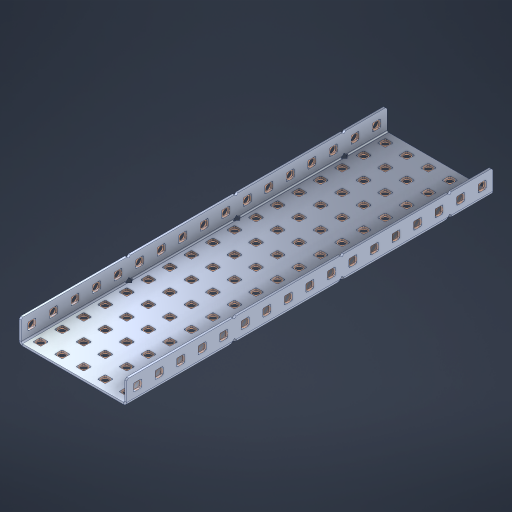
# Autodesk Inventor part: Alu C 1x3x1x35
Saved by Autodesk Inventor 2023 (Build 270158000, 158)
## iProperties
Created: 2022-07-28
Part Number: Alu C 1x3x1x35
Material: Generic
Document SubType Name: Sheet Metal
Designer: ylu12
Density: 1 g/cm^3
Sheet Metal Rule: Default
Appearance: Steel
Author: ylu12
Autodesk Inventor part; units mm, degrees
ref_plane "YZ Plane" through (0, 0, 0) normal (1, 0, 0) x (0, 1, 0)
ref_plane "XZ Plane" through (0, 0, 0) normal (0, 1, 0) x (-1, 0, 0)
sketch "Sketch1" plane through (0, 0, 0) normal (0, 1, 0) x (-1, 0, 0)
  line L0 (-31.75, 0) -> (31.75, 0)
  line L1 (31.75, 0) -> (31.75, -215.9)
  line L2 (31.75, -215.9) -> (-31.75, -215.9)
  line L3 (-31.75, -215.9) -> (-31.75, 0)
  line L4 (31.75, 0) -> (-31.75, -215.9) construction
  point P0 (0, 0)
  point P1 (0, 0)
  dimension "d0" = 63.5
  dimension "d1" = 215.9
  measures "d0" distance of L1.end L2.end
  measures "d1" distance of L0.end L1.end
extrude "Plate1" add sketch "Sketch1" along normal blind 1.1906
sketch "Sketch2" plane through (30.5594, 0, -215.9) normal (1, 0, 0) x (0, 1, 0)
  line L0 (0, 215.9) -> (0, 0)
  line L1 (0, 0) -> (13.8906, 0)
  line L2 (13.8906, 0) -> (13.8906, 215.9)
  line L3 (13.8906, 215.9) -> (0, 215.9)
  constraints: 6 end point, 1 horizontal, 1 perpendicular, 1 vertical
edge flange "Flanges" height 12.7 angle 90 thickness 1.1906 bend radius 0.7937 thickness toward (1, 0, 0) relief tear relief width 1.1906 relief depth 0.5953 corner gap 1.1906 corner form 0 edges at (31.75, 1.1906, -107.95) (-31.75, 1.1906, -107.95) wall of the first edge with corners at (30.5594, 0, 0) (30.5594, 0, -215.9) (30.5594, 13.8906, -215.9) (30.5594, 13.8906, 0)
bend "Bend1"
corner "Corner1"
sketch "Sketch3" plane through (31.75, 1.9844, -215.9) normal (1, 0, 0) x (0, 0, -1)
  line L0 (-211.3534, 7.8677) -> (-207.7466, 7.8677)
  line L1 (-207.2386, 7.3597) -> (-207.2386, 3.7529)
  line L2 (-207.7466, 3.2449) -> (-211.3534, 3.2449)
  line L3 (-211.8614, 3.7529) -> (-211.8614, 7.3597)
  arc A0 (-211.3534, 7.8677) -> (-211.8614, 7.3597) centre (-211.3534, 7.3597) ccw
  arc A1 (-207.2386, 7.3597) -> (-207.7466, 7.8677) centre (-207.7466, 7.3597) ccw
  arc A2 (-207.7466, 3.2449) -> (-207.2386, 3.7529) centre (-207.7466, 3.7529) ccw
  arc A3 (-211.8614, 3.7529) -> (-211.3534, 3.2449) centre (-211.3534, 3.7529) ccw
  line L4 (-215.9, 0) -> (-215.9, 11.9063) construction
  line L5 (-215.9, 11.9063) -> (0, 11.9063) construction
  line L6 (-211.3534, 7.3597) -> (-207.7466, 3.7529) construction
  point P0 (-215.9, -1.9844)
  point P1 (-207.2386, 3.2449)
  point P2 (-211.8614, 3.2449)
  point P3 (-209.55, 5.5563)
  dimension "d16" = 4.6228
  dimension "d17" = 0.508
  dimension "d20" = 6.35
  dimension "d21" = 6.35
  constraints: 10 end point, 8 point on circle, 8 tangent, 4 centre point, 4 point on line, 3 equal radius, 2 parallel, 2 perpendicular, 1 horizontal, 1 midpoint
  measures "d16" distance of point (-207.239, 3.245) point (-211.861, 3.245)
  measures "d17" radius of A0
  measures "d20" distance from line of point (-209.55, 5.556) L4
  measures "d21" distance from line of L5 point (-209.55, 5.556)
extrude "Flange Stamp" cut sketch "Sketch3" against normal blind 1.1906
sketch "Sketch7" plane through (31.75, 1.9844, 0) normal (1, 0, 0) x (0, 0, -1)
  arc A0 (4.5466, 7.8677) -> (4.0386, 7.3597) centre (4.5466, 7.3597) ccw construction
  arc A1 (8.1534, 3.2449) -> (8.6614, 3.7529) centre (8.1534, 3.7529) ccw construction
  circle A2 centre (6.35, 5.5563) radius 2.1844
  line L0 (4.5466, 7.3597) -> (8.1534, 3.7529) construction
  point P0 (0, -1.9844)
  dimension "d46" = 4.3688
  constraints: 2 end point, 1 centre point, 1 midpoint
  measures "d46" diameter of A2
surface extrude "Flange Circle" sketch "Sketch7" against normal up to surface (1.1906 mm away) shown yes curves A2
ref_plane "Flange Pattern Plane" through (31.75, 7.5406, -4.5466) normal (0, 1, 0) x (1, 0, 0)
pattern_sketch "Flange Pattern" of "Flange Circle", "Flange Stamp" from (31.75, 7.5406, -6.35) facing (1, 0, 0) copies at (31.75, 7.5406, -19.05) facing (1, 0, 0) at (31.75, 7.5406, -31.75) facing (1, 0, 0) at (31.75, 7.5406, -44.45) facing (1, 0, 0) at (31.75, 7.5406, -57.15) facing (1, 0, 0) at (31.75, 7.5406, -69.85) facing (1, 0, 0) at (31.75, 7.5406, -82.55) facing (1, 0, 0) at (31.75, 7.5406, -95.25) facing (1, 0, 0) at (31.75, 7.5406, -107.95) facing (1, 0, 0) at (31.75, 7.5406, -120.65) facing (1, 0, 0) at (31.75, 7.5406, -133.35) facing (1, 0, 0) at (31.75, 7.5406, -146.05) facing (1, 0, 0) at (31.75, 7.5406, -158.75) facing (1, 0, 0) at (31.75, 7.5406, -171.45) facing (1, 0, 0) at (31.75, 7.5406, -184.15) facing (1, 0, 0) at (31.75, 7.5406, -196.85) facing (1, 0, 0) at (31.75, 7.5406, -209.55) facing (1, 0, 0) at (-31.75, 7.5406, -6.35) facing (-1, 0, 0) at (-31.75, 7.5406, -19.05) facing (-1, 0, 0) at (-31.75, 7.5406, -31.75) facing (-1, 0, 0) at (-31.75, 7.5406, -44.45) facing (-1, 0, 0) at (-31.75, 7.5406, -57.15) facing (-1, 0, 0) at (-31.75, 7.5406, -69.85) facing (-1, 0, 0) at (-31.75, 7.5406, -82.55) facing (-1, 0, 0) at (-31.75, 7.5406, -95.25) facing (-1, 0, 0) at (-31.75, 7.5406, -107.95) facing (-1, 0, 0) at (-31.75, 7.5406, -120.65) facing (-1, 0, 0) at (-31.75, 7.5406, -133.35) facing (-1, 0, 0) at (-31.75, 7.5406, -146.05) facing (-1, 0, 0) at (-31.75, 7.5406, -158.75) facing (-1, 0, 0) at (-31.75, 7.5406, -171.45) facing (-1, 0, 0) at (-31.75, 7.5406, -184.15) facing (-1, 0, 0) at (-31.75, 7.5406, -196.85) facing (-1, 0, 0) at (-31.75, 7.5406, -209.55) facing (-1, 0, 0)
sketch "Sketch8" plane through (0, 0, 0) normal (0, -1, 0) x (1, 0, 0)
  line L0 (29.7656, 0) -> (-29.7656, 0) construction
  line L1 (27.2034, -4.0386) -> (23.5966, -4.0386)
  line L2 (23.0886, -4.5466) -> (23.0886, -8.1534)
  line L3 (23.5966, -8.6614) -> (27.2034, -8.6614)
  line L4 (27.7114, -8.1534) -> (27.7114, -4.5466)
  arc A0 (27.7114, -4.5466) -> (27.2034, -4.0386) centre (27.2034, -4.5466) ccw
  arc A1 (27.2034, -8.6614) -> (27.7114, -8.1534) centre (27.2034, -8.1534) ccw
  arc A2 (23.0886, -8.1534) -> (23.5966, -8.6614) centre (23.5966, -8.1534) ccw
  arc A3 (23.5966, -4.0386) -> (23.0886, -4.5466) centre (23.5966, -4.5466) ccw
  line L5 (27.2034, -4.5466) -> (23.5966, -8.1534) construction
  line L6 (31.75, 0) -> (31.75, -215.9) construction
  point P0 (0, 0)
  point P1 (23.0886, -8.6614)
  point P2 (27.7114, -8.6614)
  point P3 (25.4, -6.35)
  dimension "d49" = 4.6228
  dimension "d50" = 0.508
  dimension "d51" = 6.35
  dimension "d52" = 6.35
  constraints: 10 end point, 8 point on circle, 8 tangent, 4 centre point, 4 point on line, 3 equal radius, 2 parallel, 2 perpendicular, 1 horizontal, 1 midpoint
  measures "d49" distance of point (27.711, -8.661) point (23.089, -8.661)
  measures "d50" radius of A0
  measures "d51" distance from line of L6 point (25.4, -6.35)
  measures "d52" distance from line of L0 point (25.4, -6.35)
extrude "Body Stamp" cut sketch "Sketch8" against normal blind 1.1906
sketch "Sketch9" plane through (0, 0, 0) normal (0, -1, 0) x (1, 0, 0)
  arc A0 (27.7114, -4.5466) -> (27.2034, -4.0386) centre (27.2034, -4.5466) ccw construction
  arc A1 (23.0886, -8.1534) -> (23.5966, -8.6614) centre (23.5966, -8.1534) ccw construction
  line L0 (27.2034, -4.5466) -> (23.5966, -8.1534) construction
  circle A2 centre (25.4, -6.35) radius 2.1844
  point P0 (0, 0)
  dimension "d55" = 4.3688
  constraints: 2 end point, 1 centre point, 1 midpoint
  measures "d55" diameter of A2
surface extrude "Body Circle" sketch "Sketch9" against normal up to surface (1.1906 mm away) shown yes curves A2
pattern_sketch "Body Pattern" of "Body Stamp", "Body Circle" from (25.4, 0, -6.35) copies at (25.4, 0, -19.05) at (25.4, 0, -31.75) at (25.4, 0, -44.45) at (25.4, 0, -57.15) at (25.4, 0, -69.85) at (25.4, 0, -82.55) at (25.4, 0, -95.25) at (25.4, 0, -107.95) at (25.4, 0, -120.65) at (25.4, 0, -133.35) at (25.4, 0, -146.05) at (25.4, 0, -158.75) at (25.4, 0, -171.45) at (25.4, 0, -184.15) at (25.4, 0, -196.85) at (25.4, 0, -209.55) at (12.7, 0, -6.35) at (12.7, 0, -19.05) at (12.7, 0, -31.75) at (12.7, 0, -44.45) at (12.7, 0, -57.15) at (12.7, 0, -69.85) at (12.7, 0, -82.55) at (12.7, 0, -95.25) at (12.7, 0, -107.95) at (12.7, 0, -120.65) at (12.7, 0, -133.35) at (12.7, 0, -146.05) at (12.7, 0, -158.75) at (12.7, 0, -171.45) at (12.7, 0, -184.15) at (12.7, 0, -196.85) at (12.7, 0, -209.55) at (0, 0, -6.35) at (0, 0, -19.05) at (0, 0, -31.75) at (0, 0, -44.45) at (0, 0, -57.15) at (0, 0, -69.85) at (0, 0, -82.55) at (0, 0, -95.25) at (0, 0, -107.95) at (0, 0, -120.65) at (0, 0, -133.35) at (0, 0, -146.05) at (0, 0, -158.75) at (0, 0, -171.45) at (0, 0, -184.15) at (0, 0, -196.85) at (0, 0, -209.55) at (-12.7, 0, -6.35) at (-12.7, 0, -19.05) at (-12.7, 0, -31.75) at (-12.7, 0, -44.45) at (-12.7, 0, -57.15) at (-12.7, 0, -69.85) at (-12.7, 0, -82.55) at (-12.7, 0, -95.25) at (-12.7, 0, -107.95) at (-12.7, 0, -120.65) at (-12.7, 0, -133.35) at (-12.7, 0, -146.05) at (-12.7, 0, -158.75) at (-12.7, 0, -171.45) at (-12.7, 0, -184.15) at (-12.7, 0, -196.85) at (-12.7, 0, -209.55) at (-25.4, 0, -6.35) at (-25.4, 0, -19.05) at (-25.4, 0, -31.75) at (-25.4, 0, -44.45) at (-25.4, 0, -57.15) at (-25.4, 0, -69.85) at (-25.4, 0, -82.55) at (-25.4, 0, -95.25) at (-25.4, 0, -107.95) at (-25.4, 0, -120.65) at (-25.4, 0, -133.35) at (-25.4, 0, -146.05) at (-25.4, 0, -158.75) at (-25.4, 0, -171.45) at (-25.4, 0, -184.15) at (-25.4, 0, -196.85) at (-25.4, 0, -209.55)
sketch "Arc Length" plane through (30.5594, 1.9844, 0) normal (0, 0, 1) x (1, 0, 0)
  line L0 (0, 0) -> (1.1906, 0) construction
  arc A0 (-0.7938, -0.7938) -> (0, 0) centre (-0.7938, 0) ccw construction
  line L1 (-0.7938, -1.9844) -> (-0.7938, -0.7938) construction
  arc A1 (-0.7938, -1.9844) -> (1.1906, 0) centre (-0.7938, 0) ccw construction
  point P0 (-30.5594, -1.9844)
  dimension "d85" = 3.117
  dimension "d92" = 1.2468
sketch "Sketch13" plane through (31.75, 13.8906, 0) normal (1, 0, 0) x (0, 0, -1)
  line L0 (0, 0) -> (215.9, 0) construction
  line L1 (62.4078, 0) -> (63.4238, -1.016)
  line L2 (63.4238, -1.016) -> (64.4398, 0)
  line L3 (62.4078, 0) -> (64.4398, 0)
  line L4 (215.9, -11.9063) -> (0, -11.9063) construction
  line L5 (63.4238, -10.8903) -> (61.3168, -12.9972)
  line L6 (61.3168, -12.9972) -> (63.4238, -15.1042)
  line L7 (63.4238, -15.1042) -> (65.5308, -12.9972)
  line L8 (65.5308, -12.9972) -> (63.4238, -10.8903)
  line L9 (63.4238, -10.8903) -> (63.4238, -15.1042) construction
  line L10 (63.4238, -1.016) -> (63.4238, -10.8903) construction
  line L11 (0, -11.9063) -> (215.9, -11.9063) construction
  point P0 (0, -13.8906)
  dimension "d86" = 4.2139
  dimension "d88" = 1.016
  dimension "d91" = 1.016
  dimension "d102" = 63.4238
  constraints: 19 end point, 6 perpendicular, 2 point on line, 2 vertical, 1 collinear
  measures "d86" distance of L5.start L6.end
  measures "d88" distance from line of L0 L1.end
  measures "d91" distance from line of L5.start L11
  measures "d102" distance from line of L0.start L10
cut across bends "Notch" sketch "Sketch13" k factor 0.44
mirror "Notch Mirror" about plane through (0, 0, 0) normal (1, 0, 0) of "Notch"
pattern_linear "Notch Pattern" count 3 spacing 63.5 along (0, 0, -1) of "Notch", "Notch Mirror"
chamfer "End Chamfer" distance 1.016 angle 45 4 edges at (-31.1547, 13.8906, -215.9) (31.1547, 13.8906, -215.9) (-31.1547, 13.8906, 0) (31.1547, 13.8906, 0)
sketch "Sketch14" plane through (-31.75, 1.9844, 228.6) normal (1, 0, 0) x (0, 0, -1)
  line L0 (228.6, 11.9062) -> (444.5, 11.9062) construction
  line L1 (228.6, 0) -> (228.6, 11.9062) construction
  line L2 (228.6, -1.9844) -> (444.5, -1.9844) construction
  line L3 (228.6, 11.9062) -> (444.5, 11.9062)
  line L4 (444.5, 11.9062) -> (444.5, -1.9844)
  line L5 (444.5, -1.9844) -> (228.6, -1.9844)
  line L6 (228.6, -1.9844) -> (228.6, 11.9062)
  point P0 (382.0521, -1.9844)
  constraints: 8 end point, 2 collinear, 2 parallel, 1 horizontal, 1 perpendicular
extrude "Half Cut" [suppressed]
sketch "Flange Pattern Sketch" plane through (31.75, 7.5406, -4.5466) normal (0, 1, 0) x (1, 0, 0)
  line L0 (0, 3.6068) -> (0, 0) construction
  line L1 (-76.2822, -4.5466) -> (13.1932, -4.5466) construction
  line L2 (0, 0) -> (-1.1906, 0) construction
  point P0 (-31.75, -4.5466)
  point P1 (0, 1.8034)
  point P2 (0, 14.5034)
  point P3 (0, 27.2034)
  point P4 (0, 39.9034)
  point P5 (0, 52.6034)
  point P6 (0, 65.3034)
  point P7 (0, 78.0034)
  point P8 (0, 90.7034)
  point P9 (0, 103.4034)
  point P10 (0, 116.1034)
  point P11 (0, 128.8034)
  point P12 (0, 141.5034)
  point P13 (0, 154.2034)
  point P14 (0, 166.9034)
  point P15 (0, 179.6034)
  point P16 (0, 192.3034)
  point P17 (0, 205.0034)
  point P18 (-63.5, 1.8034)
  point P19 (-63.5, 14.5034)
  point P20 (-63.5, 27.2034)
  point P21 (-63.5, 39.9034)
  point P22 (-63.5, 52.6034)
  point P23 (-63.5, 65.3034)
  point P24 (-63.5, 78.0034)
  point P25 (-63.5, 90.7034)
  point P26 (-63.5, 103.4034)
  point P27 (-63.5, 116.1034)
  point P28 (-63.5, 128.8034)
  point P29 (-63.5, 141.5034)
  point P30 (-63.5, 154.2034)
  point P31 (-63.5, 166.9034)
  point P32 (-63.5, 179.6034)
  point P33 (-63.5, 192.3034)
  point P34 (-63.5, 205.0034)
  dimension "d131" = 63.5
  dimension "d134" = 12.7
  constraints: 1 horizontal, 1 midpoint, 1 vertical, 33 other
  measures "d134" distance of point (0, 1.803) point (0, 14.503)
sketch "Body Pattern Sketch" plane through (0, 0, 0) normal (0, -1, 0) x (1, 0, 0)
  line L0 (29.7656, 0) -> (-29.7656, 0) construction
  line L1 (31.75, 0) -> (31.75, -215.9) construction
  circle A0 centre (25.4, -6.35) radius 2.1844 construction
  point P0 (0, 0)
  point P1 (25.4, -19.05)
  point P2 (25.4, -31.75)
  point P3 (25.4, -44.45)
  point P4 (25.4, -57.15)
  point P5 (25.4, -69.85)
  point P6 (25.4, -82.55)
  point P7 (25.4, -95.25)
  point P8 (25.4, -107.95)
  point P9 (25.4, -120.65)
  point P10 (25.4, -133.35)
  point P11 (25.4, -146.05)
  point P12 (25.4, -158.75)
  point P13 (25.4, -171.45)
  point P14 (25.4, -184.15)
  point P15 (25.4, -196.85)
  point P16 (25.4, -209.55)
  point P17 (12.7, -6.35)
  point P18 (12.7, -19.05)
  point P19 (12.7, -31.75)
  point P20 (12.7, -44.45)
  point P21 (12.7, -57.15)
  point P22 (12.7, -69.85)
  point P23 (12.7, -82.55)
  point P24 (12.7, -95.25)
  point P25 (12.7, -107.95)
  point P26 (12.7, -120.65)
  point P27 (12.7, -133.35)
  point P28 (12.7, -146.05)
  point P29 (12.7, -158.75)
  point P30 (12.7, -171.45)
  point P31 (12.7, -184.15)
  point P32 (12.7, -196.85)
  point P33 (12.7, -209.55)
  point P34 (0, -6.35)
  point P35 (0, -19.05)
  point P36 (0, -31.75)
  point P37 (0, -44.45)
  point P38 (0, -57.15)
  point P39 (0, -69.85)
  point P40 (0, -82.55)
  point P41 (0, -95.25)
  point P42 (0, -107.95)
  point P43 (0, -120.65)
  point P44 (0, -133.35)
  point P45 (0, -146.05)
  point P46 (0, -158.75)
  point P47 (0, -171.45)
  point P48 (0, -184.15)
  point P49 (0, -196.85)
  point P50 (0, -209.55)
  point P51 (-12.7, -6.35)
  point P52 (-12.7, -19.05)
  point P53 (-12.7, -31.75)
  point P54 (-12.7, -44.45)
  point P55 (-12.7, -57.15)
  point P56 (-12.7, -69.85)
  point P57 (-12.7, -82.55)
  point P58 (-12.7, -95.25)
  point P59 (-12.7, -107.95)
  point P60 (-12.7, -120.65)
  point P61 (-12.7, -133.35)
  point P62 (-12.7, -146.05)
  point P63 (-12.7, -158.75)
  point P64 (-12.7, -171.45)
  point P65 (-12.7, -184.15)
  point P66 (-12.7, -196.85)
  point P67 (-12.7, -209.55)
  point P68 (-25.4, -6.35)
  point P69 (-25.4, -19.05)
  point P70 (-25.4, -31.75)
  point P71 (-25.4, -44.45)
  point P72 (-25.4, -57.15)
  point P73 (-25.4, -69.85)
  point P74 (-25.4, -82.55)
  point P75 (-25.4, -95.25)
  point P76 (-25.4, -107.95)
  point P77 (-25.4, -120.65)
  point P78 (-25.4, -133.35)
  point P79 (-25.4, -146.05)
  point P80 (-25.4, -158.75)
  point P81 (-25.4, -171.45)
  point P82 (-25.4, -184.15)
  point P83 (-25.4, -196.85)
  point P84 (-25.4, -209.55)
  dimension "d62" = 12.7
  dimension "d65" = 12.7
  dimension "d139" = 12.7
  constraints: 1 coincident, 1 horizontal, 1 vertical, 84 other
  measures "d139" distance of point (25.4, -19.05) point (25.4, -6.35)
equation "\"d1\" = 12.7 * Length"
equation "\"d18\" = Thickness"
equation "\"d53\" = Thickness"
equation "\"d10\" = CornerReliefSize"
equation "\"d89\" = Thickness"
equation "\"d2\" = Thickness"
equation "\"d3\" = BendReliefWidth"
equation "\"d4\" = BendReliefDepth"
equation "\"d5\" = MinimumRemnant"
equation "\"d6\" = TransitionRadius"
equation "\"d11\" = GapSize"
equation "\"d12\" = JacobiRadiusSize"
equation "\"BendRadius\" = Thickness"
equation "\"BendReliefWidth\" = Thickness"
equation "\"BendReliefDepth\" = 0.5 * Thickness"
equation "\"CornerReliefSize\" = 4 * Thickness"
equation "\"MinimumRemnant\" = 2 * Thickness"
equation "\"TransitionRadius\" = BendRadius"
equation "\"JacobiRadiusSize\" = BendRadius"
equation "\"GapSize\" = Thickness"
equation "\"Length\" = 17"
equation "\"Thickness\" = 1.190625"
body "Solid1"
body "Srf1"
body "Srf2"
body "Srf91"
body "Srf92"
body "Srf856"
body "Srf1310"
body "Srf1311"
body "Srf1312"
body "Srf1376"
body "Srf1377"
body "Srf1728"
body "Srf1755"
body "Srf1878"
body "Srf1879"
body "Srf1880"
body "Srf1881"
body "Srf1882"
body "Srf1883"
body "Srf1884"
body "Srf1885"
body "Srf1886"
body "Srf1887"
body "Srf1888"
body "Srf1889"
body "Srf1890"
body "Srf1891"
body "Srf1892"
body "Srf1893"
body "Srf1894"
body "Srf1895"
body "Srf1896"
body "Srf1897"
body "Srf1898"
body "Srf1899"
body "Srf1900"
body "Srf1901"
body "Srf1902"
body "Srf1903"
body "Srf1904"
body "Srf1905"
body "Srf1942"
body "Srf1943"
body "Srf1944"
body "Srf1945"
body "Srf1946"
body "Srf1947"
body "Srf1948"
body "Srf1949"
body "Srf1950"
body "Srf1951"
body "Srf1952"
body "Srf1953"
body "Srf1954"
body "Srf1955"
body "Srf1956"
body "Srf1957"
body "Srf1958"
body "Srf1959"
body "Srf1960"
body "Srf1961"
body "Srf1962"
body "Srf1963"
body "Srf1964"
body "Srf1965"
body "Srf1966"
body "Srf1967"
body "Srf1968"
body "Srf1969"
body "Srf1970"
body "Srf2146"
body "Srf2147"
body "Srf2148"
body "Srf2149"
body "Srf2150"
body "Srf2151"
body "Srf2152"
body "Srf2153"
body "Srf2154"
body "Srf2155"
body "Srf2156"
body "Srf2157"
body "Srf2158"
body "Srf2159"
body "Srf2160"
body "Srf2161"
body "Srf2162"
body "Srf2163"
body "Srf2164"
body "Srf2165"
body "Srf2166"
body "Srf2167"
body "Srf2168"
body "Srf2169"
body "Srf2170"
body "Srf2171"
body "Srf2172"
body "Srf2173"
body "Srf2174"
body "Srf2175"
body "Srf2176"
body "Srf2177"
body "Srf2178"
body "Srf2179"
body "Srf2180"
body "Srf2181"
body "Srf2182"
body "Srf2183"
body "Srf2184"
body "Srf2185"
body "Srf2186"
body "Srf2187"
body "Srf2188"
body "Srf2189"
body "Srf2190"
body "Srf2191"
body "Srf2192"
body "Srf2193"
body "Srf2194"
body "Srf2195"
